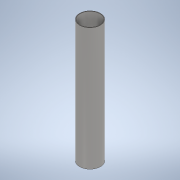
# Autodesk Inventor part: ODYSSEY-0004-001
Saved by Autodesk Inventor 2021 (Build 250183000, 183)
## iProperties
Created: 2021-08-03
Part Number: ODYSSEY-0004-001
Material: Stainless Steel, 440C
Document SubType Name: Modeling
Designer: ALEX CLAY
Density: 7.75 g/cm^3
Appearance: Semi-Polished
Mass: 138864 g
Surface Area: 37811.1 cm^2
Volume: 17918 cm^3
Project: ODYSSEY
Description: OXIDIZER TANK BARREL
Author: Alex Clay
Title: OXIDIZER TANK BARREL
Revision Number: 00
Autodesk Inventor part; units mm, degrees
ref_plane "YZ Plane" through (0, 0, 0) normal (1, 0, 0) x (0, 1, 0)
ref_plane "XZ Plane" through (0, 0, 0) normal (0, 1, 0) x (-1, 0, 0)
ref_plane "XY Plane" through (0, 0, 0) normal (0, 0, 1) x (1, 0, 0)
sketch "Sketch1" plane through (0, 0, 0) normal (0, 1, 0) x (-1, 0, 0)
  circle A0 centre (0, 0) radius 152.4
  circle A1 centre (0, 0) radius 161.925
  dimension "d0" = 323.85
  dimension "d1" = 9.525
  constraints: 2 centre point, 2 coincident
  measures "d0" diameter of A1
  measures "d1" radial gap between concentric circles of A0 A1
extrude "Extrusion1" add sketch "Sketch1" along normal blind 1905
body "Solid1"
